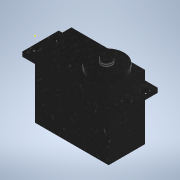
# Autodesk Inventor part: Servo
Saved by Autodesk Inventor 2021 (Build 250183000, 183)
## iProperties
Created: 2021-03-30
Part Number: Servo
Material: Oro
Document SubType Name: Modeling
Designer: diego
Density: 19.3 g/cm^3
Appearance: Textura fina - Negro
Author: diego
Autodesk Inventor part; units mm, degrees
ref_plane "YZ Plane" through (0, 0, 0) normal (1, 0, 0) x (0, 1, 0)
ref_plane "XZ Plane" through (0, 0, 0) normal (0, 1, 0) x (-1, 0, 0)
ref_plane "XY Plane" through (0, 0, 0) normal (0, 0, 1) x (1, 0, 0)
sketch "Boceto1" plane through (0, 0, 0) normal (0, 0, 1) x (1, 0, 0)
  line L0 (0, 0) -> (40.5, 0)
  line L1 (40.5, 0) -> (40.5, 28)
  line L2 (40.5, 28) -> (0, 28)
  line L3 (0, 28) -> (0, 0)
  constraints: 8 end point, 2 perpendicular, 1 horizontal, 1 vertical
extrude "Extrusión1" add sketch "Boceto1" against normal blind 20
sketch "Boceto2" plane through (0, 0, 0) normal (0, 0, 1) x (1, 0, 0)
  line L0 (0, 0) -> (0, 28) projected
  line L1 (0, 28) -> (-7, 28)
  line L2 (-7, 28) -> (-7, 30.5)
  line L3 (-7, 30.5) -> (47.5, 30.5)
  line L4 (47.5, 30.5) -> (47.5, 28)
  line L5 (40.5, 28) -> (40.5, 0) projected
  line L6 (47.5, 28) -> (40.5, 28)
  line L7 (40.5, 28) -> (0, 28)
  constraints: 12 end point, 4 perpendicular, 1 collinear, 1 horizontal, 1 point on line
extrude "Extrusión2" add sketch "Boceto2" against normal blind 20
sketch "Boceto3" plane through (0, 0, 0) normal (0, 0, 1) x (1, 0, 0)
  line L0 (0, 35.5) -> (0, 30.5)
  line L1 (47.5, 30.5) -> (-7, 30.5) projected
  line L2 (0, 30.5) -> (40.5, 30.5)
  line L3 (0, 35.5) -> (40.5, 35.5)
  line L4 (40.5, 35.5) -> (40.5, 30.5)
  point P0 (0, 0)
  constraints: 8 end point, 2 point on line, 1 horizontal, 1 perpendicular, 1 vertical
extrude "Extrusión3" add sketch "Boceto3" against normal blind 20
sketch "Boceto4" plane through (0, 35.5, 0) normal (0, 1, 0) x (1, 0, 0)
  circle A0 centre (45.5, 5.0013) radius 2
  circle A1 centre (45.5, 15.0013) radius 2
  line L0 (-7, 0) -> (-7, 20) projected
  circle A2 centre (-5, 15.0013) radius 2
  circle A3 centre (-5, 5.0013) radius 2
  point P0 (0, 0)
  constraints: 4 centre point, 2 tangent
hole "Agujero1" at (-5, 35.5, -15.0013) at (-5, 35.5, -5.0013) at (45.5, 35.5, -5.0013) at (45.5, 35.5, -15.0013) direction (0, -1, 0) diameter 4 end through all
sketch "Boceto5" plane through (0, 35.5, 0) normal (0, 1, 0) x (1, 0, 0)
  arc A0 (24.3765, 2) -> (24.3765, 18) centre (29.5, 10) ccw
  arc A1 (6.1878, 13) -> (6.1878, 7) centre (6.1878, 10) ccw
  line L0 (6.1878, 13) -> (6.1878, 15)
  line L1 (6.1878, 7) -> (6.1878, 5)
  line L2 (0, 20) -> (40.5, 20) projected
  line L3 (6.1878, 15) -> (6.1878, 18)
  line L4 (6.1878, 5) -> (6.1878, 2)
  line L5 (6.1878, 2) -> (24.3765, 2)
  line L6 (6.1878, 18) -> (24.3765, 18)
  circle A2 centre (29.5, 10) radius 9.5
  point P0 (24.3765, 18)
  point P1 (24.3765, 2)
  point P2 (24.3765, 2)
  point P3 (24.3765, 18)
  constraints: 12 end point, 4 point on circle, 4 vertical, 3 centre point, 1 coincident, 1 concentric, 1 parallel, 1 perpendicular
extrude "Extrusión4" add sketch "Boceto5" along normal blind 3 contours A2 A0
extrude "Extrusión5" add sketch "Boceto5" along normal blind 2 contours L5 L4 L1 A1 L0 L3 L6 A2
sketch "Boceto6" plane through (29.5, 38.5, -10) normal (0, 1, 0) x (1, 0, 0)
  circle A0 centre (0, 0) radius 3
  point P0 (-29.5, -10)
  constraints: 1 centre point
extrude "Extrusión6" add sketch "Boceto6" along normal blind 3
thread "Rosca1" size "M6x1" class "6g" standard "ANSI Metric M Profile" length 2
sketch "Boceto7" plane through (29.5, 41.5, -10) normal (0, 1, 0) x (1, 0, 0)
  point P0 (-29.5, -10)
